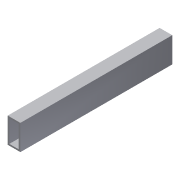
# Autodesk Inventor part: Aluminum Box Tube
Saved by Autodesk Inventor 2013 (Build 170138000, 138)
## iProperties
Created: 2012-11-10
Part Number: Aluminum Box Tube
Material: Aluminum 6061
Document SubType Name: Modeling
Designer: Nemo
Mass: 366.374 g
Surface Area: 860.482 cm^2
Volume: 135.193 cm^3
Density: 2.71 g/cm^3
Author: Nemo
Autodesk Inventor part; units mm, degrees
ref_plane "YZ Plane" through (0, 0, 0) normal (1, 0, 0) x (0, 1, 0)
ref_plane "XZ Plane" through (0, 0, 0) normal (0, 1, 0) x (-1, 0, 0)
ref_plane "XY Plane" through (0, 0, 0) normal (0, 0, 1) x (1, 0, 0)
sketch "Sketch1" plane through (0, 0, 0) normal (0, 0, 1) x (1, 0, 0)
  line L0 (-12.7, 25.4) -> (12.7, 25.4)
  line L1 (12.7, 25.4) -> (12.7, -25.4)
  line L2 (12.7, -25.4) -> (-12.7, -25.4)
  line L3 (-12.7, -25.4) -> (-12.7, 25.4)
  line L4 (9.525, 22.225) -> (-9.525, 22.225)
  line L5 (-9.525, 22.225) -> (-9.525, -22.225)
  line L6 (-9.525, -22.225) -> (9.525, -22.225)
  line L7 (9.525, -22.225) -> (9.525, 22.225)
  point P0 (0, 0)
  point P1 (0, 25.4)
  point P2 (-12.7, 0)
  constraints: 16 end point, 5 parallel, 2 horizontal alignment, 2 midpoint, 2 perpendicular, 2 vertical alignment, 1 horizontal, 3 other
extrude "Extrusion1" add sketch "Sketch1" along normal mid plane 304.8
body "Solid1"
